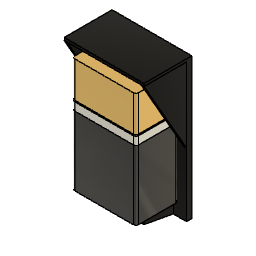
9V_battery_compartment (Autodesk Fusion 360 design; units mm, degrees)
Autodesk Fusion 360 part; units mm, degrees
sketch "Battery Body" plane through (0, 0, 0) normal (0, 0, 1) x (1, 0, 0)
  line L0 (0, 0) -> (24, 0)
  line L1 (24, 0) -> (24, 16)
  line L2 (24, 16) -> (0, 16)
  line L3 (0, 16) -> (0, 0)
  dimension "d1" = 24
  dimension "d2" = 16
  constraint horizontal L0
  constraint vertical L1
  constraint horizontal L2
  constraint vertical L3
  constraint coincident L0.start L3.end
  measures "d1" distance of L0.start L0.end
  measures "d2" distance of L0.end L1.end
extrude "Extrude1" add sketch "Battery Body" along normal blind 26 makes body 1
extrude "Extrude2" add 1 faces at (8, 10.6667, 26) along direction (0, 0, 1) blind 3 separate body on bodies 1 makes body 2
extrude "Extrude3" add 1 faces at (8, 10.6667, 29) along direction (0, 0, 1) blind 0.5 separate body on bodies 2 makes body 3
extrude "Extrude4" add 1 faces at (8, 10.6667, 29.5) along direction (0, 0, 1) blind 13.5 separate body on bodies 3 makes body 4
fillet "Fillet1" radius 1 16 edges at (0, 0, 13) (24, 0, 13) (24, 16, 13) (0, 16, 13) (0, 0, 27.5) (24, 0, 27.5) (24, 16, 27.5) (0, 16, 27.5) (0, 0, 29.25) (24, 0, 29.25) (24, 16, 29.25) (0, 16, 29.25) (0, 0, 36.25) (24, 0, 36.25) (24, 16, 36.25) (0, 16, 36.25) on bodies 1 2 3 4
sketch "Battery Terminals" plane through (0, 0, 43) normal (0, 0, 1) x (-1, 0, 0)
  arc A0 (-1, -16) -> (0, -15) centre (-1, -15) ccw
  line L0 (0, -15) -> (0, -1)
  arc A1 (0, -1) -> (-1, 0) centre (-1, -1) ccw
  line L1 (-1, 0) -> (-23, 0)
  arc A2 (-23, 0) -> (-24, -1) centre (-23, -1) ccw
  line L2 (-24, -1) -> (-24, -15)
  arc A3 (-24, -15) -> (-23, -16) centre (-23, -15) ccw
  line L3 (-23, -16) -> (-1, -16)
  circle A4 centre (-6, -8) radius 3
  circle A5 centre (-18, -8) radius 2
  circle A6 centre (-18, -8) radius 3
  circle A7 centre (-6, -8) radius 4
  dimension "d13" = 4
  dimension "d14" = 6
  dimension "d15" = 6
  dimension "d16" = 8
  dimension "d17" = 8
  dimension "d18" = 8
  dimension "d19" = 6
  dimension "d20" = 6
  constraint concentric A5 A6
  constraint concentric A4 A7
  measures "d13" diameter of A5
  measures "d14" diameter of A6
  measures "d15" diameter of A4
  measures "d16" diameter of A7
  measures "d17" distance of L1 A5.centre
  measures "d18" distance of L1 A4.centre
  measures "d19" distance of L0 A4.centre
  measures "d20" distance of L2 A5.centre
extrude "Extrude5" add sketch "Battery Terminals" along normal blind 4 separate body contours A6 | A7 makes body 5 at (15.0149, 8.2987, 44.3333) makes body 6 at (2.0199, 8.3983, 44.3333)
sketch "Battery Compartment" plane through (0, 0, 0) normal (0, 1, 0) x (1, 0, 0)
  line L0 (40, 0) -> (70, 0)
  line L1 (70, 0) -> (70, -53)
  line L2 (70, -53) -> (40, -53)
  line L3 (40, -53) -> (40, 0)
  dimension "d25" = 30
  dimension "d26" = 53
  constraint horizontal L0
  constraint vertical L1
  constraint horizontal L2
  constraint vertical L3
  measures "d25" distance of L0.start L0.end
  measures "d26" distance of L0.end L1.end
extrude "Extrude1'" add sketch "Battery Compartment" against normal blind 2 separate body makes body 7 in component "9V Battey Compartment"
sketch "Battery Compartment Fins" plane through (0, -2, 0) normal (0, -1, 0) x (1, 0, 0)
  line L0 (70, 53) -> (40, 53)
  line L1 (40, 53) -> (40, 0)
  line L2 (40, 0) -> (70, 0)
  line L3 (70, 0) -> (70, 53)
  line L4 (40, 53) -> (41, 53)
  line L5 (41, 53) -> (41, 24)
  line L6 (41, 24) -> (40, 24)
  line L7 (40, 24) -> (40, 53)
  line L8 (41, 53) -> (70, 53)
  line L9 (70, 53) -> (70, 52)
  line L10 (70, 52) -> (41, 52)
  line L11 (41, 52) -> (41, 53)
  line L12 (70, 52) -> (69, 52)
  line L13 (69, 52) -> (69, 24)
  line L14 (69, 24) -> (70, 24)
  line L15 (70, 24) -> (70, 52)
  line L16 (45, 0) -> (65, 0)
  line L17 (65, 0) -> (65, 3)
  line L18 (65, 3) -> (45, 3)
  line L19 (45, 3) -> (45, 0)
  dimension "d29" = 1
  dimension "d30" = 1
  dimension "d31" = 1
  dimension "d32" = 28
  dimension "d33" = 3
  dimension "d34" = 20
  dimension "d35" = 5
  constraint horizontal L4
  constraint vertical L5
  constraint horizontal L6
  constraint vertical L7
  constraint coincident L0.end L1.start
  constraint horizontal L8
  constraint vertical L9
  constraint horizontal L10
  constraint vertical L11
  constraint coincident L3 L9.end
  constraint horizontal L12
  constraint vertical L13
  constraint horizontal L14
  constraint vertical L15
  constraint collinear L6 L14
  constraint horizontal L16
  constraint vertical L17
  constraint horizontal L18
  constraint vertical L19
  constraint coincident L2 L16.start
  measures "d29" distance of L5.end L6.end
  measures "d30" distance of L13 L15
  measures "d31" distance of L8 L10
  measures "d32" distance of L9.end L14.end
  measures "d33" distance of L16.end L17.end
  measures "d34" distance of L16.start L16.end
  measures "d35" distance of L1 L19
extrude "Extrude2'" add sketch "Battery Compartment Fins" along normal blind 16 contours L0 L3 L5 L8 L9 L10 L11 L12 | L0 L1 L4 L5 L6 L7 L11 | L3 L10 L12 L13 L14 L15 bodies 7 in component "9V Battey Compartment"
chamfer "Chamfer1" distance 28 distance2 16 2 edges at (69.5, -18, 24) (40.5, -18, 24) measured on face at (50.3333, -18, 52.6667) measured on face at (50.3333, -18, 52.6667) on bodies 7 in component "9V Battey Compartment"
extrude "Extrude3'" add sketch "Battery Compartment Fins" along normal blind 11 contours L2 L16 L17 L18 L19 bodies 7 in component "9V Battey Compartment"
chamfer "Chamfer2" distance 2 distance2 11 1 edges at (55, -13, 0) measured on face at (58.3333, -13, 1) on bodies 7 in component "9V Battey Compartment"
sketch "Compartment Terminals" plane through (0, 0, 52) normal (0, 0, -1) x (1, 0, 0)
  line L0 (41, 2) -> (69, 2)
  line L1 (69, 2) -> (69, 18)
  line L2 (69, 18) -> (41, 18)
  line L3 (41, 18) -> (41, 2)
  circle A0 centre (49, 10) radius 3
  circle A1 centre (61, 10) radius 4
  circle A2 centre (61, 10) radius 3
  circle A3 centre (49, 10) radius 2
  line L4 (70, 2) -> (41, 2)
  dimension "d44" = 12
  dimension "d45" = 6
  dimension "d46" = 8
  dimension "d47" = 4
  dimension "d48" = 6
  dimension "d49" = 8
  dimension "d51" = 8
  dimension "d52" = 8
  constraint concentric A1 A2
  constraint concentric A0 A3
  measures "d44" distance of A0.centre A1.centre
  measures "d45" diameter of A2
  measures "d46" diameter of A1
  measures "d47" diameter of A3
  measures "d48" diameter of A0
  measures "d49" distance of A0.centre L4
  measures "d51" distance of A1.centre L4
  measures "d52" distance of L3 A0.centre
extrude "Extrude6" add sketch "Compartment Terminals" along normal blind 4 separate body contours A0 | A1 makes body 8 at (51.9851, -9.7013, 50.6667) makes body 9 at (64.9801, -9.6017, 50.6667)
fillet "Fillet3" radius 0.5 4 edges at (46.203, -8.9152, 48) (47.1353, -10.7232, 48) (58.203, -11.0848, 48) (57.2707, -8.5535, 48) on bodies 8 9
copy_body "CutPasteBodies1" bodies 9 removing the originals makes body 10 in component "9V Battey Compartment"
copy_body "CutPasteBodies2" bodies 8 removing the originals makes body 11 in component "9V Battey Compartment"
copy_body "Body->Comp1" bodies 1 removing the originals makes body 12 in component "9V Battery"
copy_body "CutPasteBodies1'" bodies 2 removing the originals makes body 13 in component "9V Battery"
copy_body "CutPasteBodies2'" bodies 3 removing the originals makes body 14 in component "9V Battery"
copy_body "CutPasteBodies3" bodies 4 removing the originals makes body 15 in component "9V Battery"
copy_body "CutPasteBodies4" bodies 5 removing the originals makes body 16 in component "9V Battery"
copy_body "CutPasteBodies5" bodies 6 removing the originals makes body 17 in component "9V Battery"
fillet "Fillet1'" radius 0.5 4 edges at (20.797, 9.0848, 47) (19.8647, 7.2768, 47) (8.797, 6.9152, 47) (9.7293, 9.4465, 47) on bodies 16 17 in component "9V Battery"
sketch "Compartment Bottom Fin Round Part" plane through (25, 0, 0) normal (1, 0, 0) x (0, 1, 0)
  line L0 (-11, 2) -> (0, 0)
  line L1 (0, 0) -> (0, 3)
  line L2 (0, 3) -> (-11, 3)
  line L3 (-11, 3) -> (-11, 2)
  ellipse E0 centre (-9, 3) end of major axis (-9, 2.5) minor radius 2
  line L4 (-9, 3.5) -> (-9, 2.5)
  line L5 (-11, 3) -> (-7, 3)
  dimension "d66" = 4
  dimension "d67" = 2
  constraint coincident L2 E0.centre
  constraint perpendicular L2 L4
  constraint coincident E0 L4.start
  constraint coincident E0 L4.end
  constraint coincident E0 L2.end
  constraint coincident E0 L5.end
  measures "d67" distance of L2.end E0.centre
extrude "Extrude4'" add sketch "Compartment Bottom Fin Round Part" against normal blind 20 contours L2 E0 L4 L5 | L2 E0 L4 L5 picked at (-9.3333, 3.311) picked at (-7.9626, 3.1385) sketch seen with x (1, 0, 0) y (0, 1, 0) z (0, 0, 1) at (40, -2, 0) bodies 7 in component "9V Battey Compartment"
component "9V Battey Compartment" placed x (1, 0, 0) y (0, 1, 0) z (0, 0, 1) at (-40, 2, 0)
component "9V Battery" placed x (1, 0, 0) y (0, 1, 0) z (0, 0, 1) at (3, -16, 5)
named bodies: "Battery Body Bottom Black Part", "Battery Body Silver Part", "Battery Body Middle Black Stripe", "Battery Body Top Brass Part", "Battery Terminal Positive", "Battery Terminal Negative", "Battery Compartment", "Compartment Terminal Negative", "Compartment Terminal Positive"
